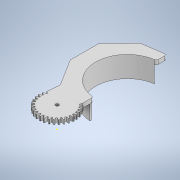
# Autodesk Inventor part: Gripper test sebelah
Saved by Autodesk Inventor 2021 (Build 250183000, 183)
## iProperties
Created: 2025-08-29
Part Number: Gripper test sebelah
Material: Generic
Document SubType Name: Modeling
Designer: Naufal K
Mass: 10.2864 g
Surface Area: 64.4788 cm^2
Volume: 10.2864 cm^3
Density: 1 g/cm^3
Appearance: Default
Author: Naufal K
Autodesk Inventor part; units mm, degrees
ref_plane "YZ Plane" through (0, 0, 0) normal (1, 0, 0) x (0, 1, 0)
ref_plane "XZ Plane" through (0, 0, 0) normal (0, 1, 0) x (-1, 0, 0)
ref_plane "XY Plane" through (0, 0, 0) normal (0, 0, 1) x (1, 0, 0)
sketch "Sketch1" plane through (0, 0, 0) normal (0, 1, 0) x (-1, 0, 0)
  arc A0 (-17.5, 0) -> (-15.9835, -7.1258) centre (0, 0) ccw
  line L0 (14.9666, 1) -> (17.4123, 0.5159)
  line L1 (17.4123, -0.5159) -> (14.9666, -1)
  line L2 (17.4929, 0.4179) -> (17.4929, -0.4179)
  line L3 (17.5, 0) -> (17.4929, 0)
  arc A1 (17.4929, 0.4179) -> (17.4123, 0.5159) centre (17.3929, 0.4179) ccw
  arc A2 (17.4123, -0.5159) -> (17.4929, -0.4179) centre (17.3929, -0.4179) ccw
  line L4 (14.459, 3.9923) -> (16.952, 4.0105)
  arc A3 (17.0507, 3.9306) -> (16.952, 4.0105) centre (16.9527, 3.9105) ccw
  line L5 (17.0507, 3.9306) -> (17.2189, 3.112)
  arc A4 (17.1597, 2.9997) -> (17.2189, 3.112) centre (17.1209, 3.0919) ccw
  line L6 (17.1597, 2.9997) -> (14.8616, 2.0332)
  line L7 (13.3593, 6.8211) -> (15.7977, 7.3408)
  arc A5 (15.9104, 7.2824) -> (15.7977, 7.3408) centre (15.8185, 7.243) ccw
  line L8 (15.9104, 7.2824) -> (16.24, 6.5144)
  arc A6 (16.2046, 6.3925) -> (16.24, 6.5144) centre (16.1481, 6.475) ccw
  line L9 (16.2046, 6.3925) -> (14.1481, 4.9832)
  line L10 (11.7128, 9.3707) -> (13.9966, 10.3705)
  arc A7 (14.1188, 10.3361) -> (13.9966, 10.3705) centre (14.0367, 10.2789) ccw
  line L11 (14.1188, 10.3361) -> (14.5962, 9.6502)
  arc A8 (14.5861, 9.5236) -> (14.5962, 9.6502) centre (14.5141, 9.593) ccw
  line L12 (14.5861, 9.5236) -> (12.8553, 7.7292)
  line L13 (9.5867, 11.5367) -> (11.6225, 12.9758)
  arc A9 (11.7491, 12.9666) -> (11.6225, 12.9758) centre (11.6802, 12.8941) ccw
  line L14 (11.7491, 12.9666) -> (12.3549, 12.3908)
  arc A10 (12.3704, 12.2648) -> (12.3549, 12.3908) centre (12.286, 12.3183) ccw
  line L15 (12.3704, 12.2648) -> (11.0363, 10.1587)
  line L16 (7.0682, 13.2303) -> (8.7726, 15.0497)
  arc A11 (8.8985, 15.0662) -> (8.7726, 15.0497) centre (8.8456, 14.9814) ccw
  line L17 (8.8985, 15.0662) -> (9.6077, 14.6242)
  arc A12 (9.6483, 14.5039) -> (9.6077, 14.6242) centre (9.5548, 14.5393) ccw
  line L18 (9.6483, 14.5039) -> (8.7655, 12.1724)
  line L19 (4.2602, 14.3823) -> (5.5635, 16.5076)
  arc A13 (5.6835, 16.5491) -> (5.5635, 16.5076) centre (5.6488, 16.4553) ccw
  line L20 (5.6835, 16.5491) -> (6.4672, 16.2588)
  arc A14 (6.5312, 16.1492) -> (6.4672, 16.2588) centre (6.4325, 16.1651) ccw
  line L21 (6.5312, 16.1492) -> (6.1357, 13.6877)
  line L22 (1.2779, 14.9455) -> (2.1267, 17.2896)
  arc A15 (2.2359, 17.3544) -> (2.1267, 17.2896) centre (2.2207, 17.2556) ccw
  line L23 (2.2359, 17.3544) -> (3.0619, 17.2279)
  arc A16 (3.1467, 17.1333) -> (3.0619, 17.2279) centre (3.0468, 17.129) ccw
  line L24 (3.1467, 17.1333) -> (3.2548, 14.6426)
  line L25 (-1.7568, 14.8968) -> (-1.3972, 17.3638)
  arc A17 (-1.3033, 17.4492) -> (-1.3972, 17.3638) centre (-1.2982, 17.3494) ccw
  line L26 (-1.3033, 17.4492) -> (-0.4687, 17.4916)
  arc A18 (-0.3666, 17.4161) -> (-0.4687, 17.4916) centre (-0.4636, 17.3917) ccw
  line L27 (-0.3666, 17.4161) -> (0.2407, 14.9981)
  line L28 (-4.7195, 14.2382) -> (-4.8639, 16.7271)
  arc A19 (-4.7891, 16.8297) -> (-4.8639, 16.7271) centre (-4.7641, 16.7329) ccw
  line L29 (-4.7891, 16.8297) -> (-3.9801, 17.0392)
  arc A20 (-3.865, 16.9857) -> (-3.9801, 17.0392) centre (-3.955, 16.9424) ccw
  line L30 (-3.865, 16.9857) -> (-2.7833, 14.7395)
  line L31 (-7.489, 12.9967) -> (-8.1315, 15.4056)
  arc A21 (-8.0789, 15.5211) -> (-8.1315, 15.4056) centre (-8.0349, 15.4314) ccw
  line L32 (-8.0789, 15.5211) -> (-7.3286, 15.8892)
  arc A22 (-7.205, 15.86) -> (-7.3286, 15.8892) centre (-7.2846, 15.7994) ccw
  line L33 (-7.205, 15.86) -> (-5.6934, 13.8775)
  line L34 (-9.9519, 11.2231) -> (-11.0662, 13.4534)
  arc A23 (-11.0379, 13.5772) -> (-11.0662, 13.4534) centre (-10.9767, 13.4981) ccw
  line L35 (-11.0379, 13.5772) -> (-10.3771, 14.0887)
  arc A24 (-10.2502, 14.085) -> (-10.3771, 14.0887) centre (-10.3158, 14.0096) ccw
  line L36 (-10.2502, 14.085) -> (-8.3704, 12.4474)
  line L37 (-12.0074, 8.9901) -> (-13.5478, 10.9504)
  arc A25 (-13.545, 11.0773) -> (-13.5478, 10.9504) centre (-13.4691, 11.0122) ccw
  line L38 (-13.545, 11.0773) -> (-13.0007, 11.7114)
  arc A26 (-12.8756, 11.7334) -> (-13.0007, 11.7114) centre (-12.9248, 11.6463) ccw
  line L39 (-12.8756, 11.7334) -> (-10.7047, 10.5076)
  line L40 (-13.5713, 6.389) -> (-15.4748, 7.9991)
  arc A27 (-15.4976, 8.124) -> (-15.4748, 7.9991) centre (-15.4102, 8.0754) ccw
  line L41 (-15.4976, 8.124) -> (-15.092, 8.8547)
  arc A28 (-14.974, 8.9013) -> (-15.092, 8.8547) centre (-15.0046, 8.8061) ccw
  line L42 (-14.974, 8.9013) -> (-12.6007, 8.1377)
  line L43 (-14.5796, 3.5263) -> (-16.7682, 4.7203)
  arc A29 (-16.8157, 4.838) -> (-16.7682, 4.7203) centre (-16.7203, 4.8081) ccw
  line L44 (-16.8157, 4.838) -> (-16.5655, 5.6354)
  arc A30 (-16.4593, 5.7049) -> (-16.5655, 5.6354) centre (-16.4701, 5.6055) ccw
  line L45 (-16.4593, 5.7049) -> (-13.9809, 5.4346)
  line L46 (-14.991, 0.5193) -> (-17.3751, 1.2483)
  arc A31 (-17.4454, 1.354) -> (-17.3751, 1.2483) centre (-17.3459, 1.3439) ccw
  line L47 (-17.4454, 1.354) -> (-17.3608, 2.1854)
  arc A32 (-17.2707, 2.2749) -> (-17.3608, 2.1854) centre (-17.2613, 2.1753) ccw
  line L48 (-17.2707, 2.2749) -> (-14.7887, 2.509)
  line L49 (-14.7887, -2.509) -> (-17.2707, -2.2749)
  arc A33 (-17.3608, -2.1854) -> (-17.2707, -2.2749) centre (-17.2613, -2.1753) ccw
  line L50 (-17.3608, -2.1854) -> (-17.4454, -1.354)
  arc A34 (-17.3751, -1.2483) -> (-17.4454, -1.354) centre (-17.3459, -1.3439) ccw
  line L51 (-17.3751, -1.2483) -> (-14.991, -0.5193)
  line L52 (-13.9809, -5.4346) -> (-16.4593, -5.7049)
  arc A35 (-16.5655, -5.6354) -> (-16.4593, -5.7049) centre (-16.4701, -5.6055) ccw
  line L53 (-16.5655, -5.6354) -> (-16.8157, -4.838)
  arc A36 (-16.7682, -4.7203) -> (-16.8157, -4.838) centre (-16.7203, -4.8081) ccw
  line L54 (-16.7682, -4.7203) -> (-14.5796, -3.5263)
  line L55 (-12.6007, -8.1377) -> (-14.974, -8.9013)
  arc A37 (-15.092, -8.8547) -> (-14.974, -8.9013) centre (-15.0046, -8.8061) ccw
  line L56 (-15.092, -8.8547) -> (-15.4976, -8.124)
  arc A38 (-15.4748, -7.9991) -> (-15.4976, -8.124) centre (-15.4102, -8.0754) ccw
  line L57 (-15.4748, -7.9991) -> (-13.5713, -6.389)
  line L58 (-10.7047, -10.5076) -> (-12.8756, -11.7334)
  arc A39 (-13.0007, -11.7114) -> (-12.8756, -11.7334) centre (-12.9248, -11.6463) ccw
  line L59 (-13.0007, -11.7114) -> (-13.545, -11.0773)
  arc A40 (-13.5478, -10.9504) -> (-13.545, -11.0773) centre (-13.4691, -11.0122) ccw
  line L60 (-13.5478, -10.9504) -> (-12.0074, -8.9901)
  line L61 (-8.3704, -12.4474) -> (-10.2502, -14.085)
  arc A41 (-10.3771, -14.0887) -> (-10.2502, -14.085) centre (-10.3158, -14.0096) ccw
  line L62 (-10.3771, -14.0887) -> (-11.0379, -13.5772)
  arc A42 (-11.0662, -13.4534) -> (-11.0379, -13.5772) centre (-10.9767, -13.4981) ccw
  line L63 (-11.0662, -13.4534) -> (-9.9519, -11.2231)
  line L64 (-5.6934, -13.8775) -> (-7.205, -15.86)
  arc A43 (-7.3286, -15.8892) -> (-7.205, -15.86) centre (-7.2846, -15.7994) ccw
  line L65 (-7.3286, -15.8892) -> (-8.0789, -15.5211)
  arc A44 (-8.1315, -15.4056) -> (-8.0789, -15.5211) centre (-8.0349, -15.4314) ccw
  line L66 (-8.1315, -15.4056) -> (-7.489, -12.9967)
  line L67 (-2.7833, -14.7395) -> (-3.865, -16.9857)
  arc A45 (-3.9801, -17.0392) -> (-3.865, -16.9857) centre (-3.955, -16.9424) ccw
  line L68 (-3.9801, -17.0392) -> (-4.7891, -16.8297)
  arc A46 (-4.8639, -16.7271) -> (-4.7891, -16.8297) centre (-4.7641, -16.7329) ccw
  line L69 (-4.8639, -16.7271) -> (-4.7195, -14.2382)
  line L70 (0.2407, -14.9981) -> (-0.3666, -17.4161)
  arc A47 (-0.4687, -17.4916) -> (-0.3666, -17.4161) centre (-0.4636, -17.3917) ccw
  line L71 (-0.4687, -17.4916) -> (-1.3033, -17.4492)
  arc A48 (-1.3972, -17.3638) -> (-1.3033, -17.4492) centre (-1.2982, -17.3494) ccw
  line L72 (-1.3972, -17.3638) -> (-1.7568, -14.8968)
  line L73 (3.2548, -14.6426) -> (3.1467, -17.1333)
  arc A49 (3.0619, -17.2279) -> (3.1467, -17.1333) centre (3.0468, -17.129) ccw
  line L74 (3.0619, -17.2279) -> (2.2359, -17.3544)
  arc A50 (2.1267, -17.2896) -> (2.2359, -17.3544) centre (2.2207, -17.2556) ccw
  line L75 (2.1267, -17.2896) -> (1.2779, -14.9455)
  line L76 (6.1357, -13.6877) -> (6.5312, -16.1492)
  arc A51 (6.4672, -16.2588) -> (6.5312, -16.1492) centre (6.4325, -16.1651) ccw
  line L77 (6.4672, -16.2588) -> (5.6835, -16.5491)
  arc A52 (5.5635, -16.5076) -> (5.6835, -16.5491) centre (5.6488, -16.4553) ccw
  line L78 (5.5635, -16.5076) -> (4.2602, -14.3823)
  line L79 (8.7655, -12.1724) -> (9.6483, -14.5039)
  arc A53 (9.6077, -14.6242) -> (9.6483, -14.5039) centre (9.5548, -14.5393) ccw
  line L80 (9.6077, -14.6242) -> (8.8985, -15.0662)
  arc A54 (8.7726, -15.0497) -> (8.8985, -15.0662) centre (8.8456, -14.9814) ccw
  line L81 (8.7726, -15.0497) -> (7.0682, -13.2303)
  line L82 (11.0363, -10.1587) -> (12.3704, -12.2648)
  arc A55 (12.3549, -12.3908) -> (12.3704, -12.2648) centre (12.286, -12.3183) ccw
  line L83 (12.3549, -12.3908) -> (11.7491, -12.9666)
  arc A56 (11.6225, -12.9758) -> (11.7491, -12.9666) centre (11.6802, -12.8941) ccw
  line L84 (11.6225, -12.9758) -> (9.5867, -11.5367)
  line L85 (12.8553, -7.7292) -> (14.5861, -9.5236)
  arc A57 (14.5962, -9.6502) -> (14.5861, -9.5236) centre (14.5141, -9.593) ccw
  line L86 (14.5962, -9.6502) -> (14.1188, -10.3361)
  arc A58 (13.9966, -10.3705) -> (14.1188, -10.3361) centre (14.0367, -10.2789) ccw
  line L87 (13.9966, -10.3705) -> (11.7128, -9.3707)
  line L88 (14.1481, -4.9832) -> (16.2046, -6.3925)
  arc A59 (16.24, -6.5144) -> (16.2046, -6.3925) centre (16.1481, -6.475) ccw
  line L89 (16.24, -6.5144) -> (15.9104, -7.2824)
  arc A60 (15.7977, -7.3408) -> (15.9104, -7.2824) centre (15.8185, -7.243) ccw
  line L90 (15.7977, -7.3408) -> (13.3593, -6.8211)
  line L91 (14.8616, -2.0332) -> (17.1597, -2.9997)
  arc A61 (17.2189, -3.112) -> (17.1597, -2.9997) centre (17.1209, -3.0919) ccw
  line L92 (17.2189, -3.112) -> (17.0507, -3.9306)
  arc A62 (16.952, -4.0105) -> (17.0507, -3.9306) centre (16.9527, -3.9105) ccw
  line L93 (16.952, -4.0105) -> (14.459, -3.9923)
  arc A63 (14.459, 3.9923) -> (14.1481, 4.9832) centre (0, 0) ccw
  arc A64 (13.3593, 6.8211) -> (12.8553, 7.7292) centre (0, 0) ccw
  arc A65 (11.7128, 9.3707) -> (11.0363, 10.1587) centre (0, 0) ccw
  arc A66 (9.5867, 11.5367) -> (8.7655, 12.1724) centre (0, 0) ccw
  arc A67 (7.0682, 13.2303) -> (6.1357, 13.6877) centre (0, 0) ccw
  arc A68 (4.2602, 14.3823) -> (3.2548, 14.6426) centre (0, 0) ccw
  arc A69 (1.2779, 14.9455) -> (0.2407, 14.9981) centre (0, 0) ccw
  arc A70 (-1.7568, 14.8968) -> (-2.7833, 14.7395) centre (0, 0) ccw
  arc A71 (-4.7195, 14.2382) -> (-5.6934, 13.8775) centre (0, 0) ccw
  arc A72 (-7.489, 12.9967) -> (-8.3704, 12.4474) centre (0, 0) ccw
  arc A73 (-9.9519, 11.2231) -> (-10.7047, 10.5076) centre (0, 0) ccw
  arc A74 (-12.0074, 8.9901) -> (-12.6007, 8.1377) centre (0, 0) ccw
  arc A75 (-13.5713, 6.389) -> (-13.9809, 5.4346) centre (0, 0) ccw
  arc A76 (-14.5796, 3.5263) -> (-14.7887, 2.509) centre (0, 0) ccw
  arc A77 (-14.991, 0.5193) -> (-14.991, -0.5193) centre (0, 0) ccw
  arc A78 (-14.7887, -2.509) -> (-14.5796, -3.5263) centre (0, 0) ccw
  arc A79 (-13.9809, -5.4346) -> (-13.5713, -6.389) centre (0, 0) ccw
  arc A80 (-12.6007, -8.1377) -> (-12.0074, -8.9901) centre (0, 0) ccw
  arc A81 (-10.7047, -10.5076) -> (-9.9519, -11.2231) centre (0, 0) ccw
  arc A82 (-8.3704, -12.4474) -> (-7.489, -12.9967) centre (0, 0) ccw
  arc A83 (-5.6934, -13.8775) -> (-4.7195, -14.2382) centre (0, 0) ccw
  arc A84 (-2.7833, -14.7395) -> (-1.7568, -14.8968) centre (0, 0) ccw
  arc A85 (0.2407, -14.9981) -> (1.2779, -14.9455) centre (0, 0) ccw
  arc A86 (3.2548, -14.6426) -> (4.2602, -14.3823) centre (0, 0) ccw
  arc A87 (6.1357, -13.6877) -> (7.0682, -13.2303) centre (0, 0) ccw
  arc A88 (8.7655, -12.1724) -> (9.5867, -11.5367) centre (0, 0) ccw
  arc A89 (11.0363, -10.1587) -> (11.7128, -9.3707) centre (0, 0) ccw
  arc A90 (12.8553, -7.7292) -> (13.3593, -6.8211) centre (0, 0) ccw
  arc A91 (14.1481, -4.9832) -> (14.459, -3.9923) centre (0, 0) ccw
  arc A92 (14.8616, -2.0332) -> (14.9666, -1) centre (0, 0) ccw
  arc A93 (14.9666, 1) -> (14.8616, 2.0332) centre (0, 0) ccw
  arc A94 (-10.7047, -83.8219) -> (-10.7047, -23.8219) centre (-10.7047, -53.8219) ccw
  line L94 (-10.7047, -83.8219) -> (-10.7047, -93.8219)
  line L95 (-10.7047, -93.8219) -> (11.3814, -90.5076)
  line L96 (11.3814, -90.5076) -> (30.7761, -70.2991)
  line L97 (30.7761, -70.2991) -> (30.7761, -43.252)
  line L98 (30.7761, -43.252) -> (14.923, -18.0076)
  line L99 (14.923, -18.0076) -> (15.9104, -7.2824)
  line L100 (-10.7047, -23.8219) -> (-10.7047, -10.5076)
  point P0 (17.1348, 3.5213)
  point P1 (-14.2219, -10.1974)
  point P2 (16.0752, 6.8984)
  point P3 (-11.8781, -12.8515)
  point P4 (14.3575, 9.9931)
  point P5 (-9.048, -14.9795)
  point P6 (12.052, 12.6787)
  point P7 (-5.8474, -16.4942)
  point P8 (9.2531, 14.8452)
  point P9 (-2.4075, -17.3336)
  point P10 (6.0754, 16.404)
  point P11 (1.131, -17.4634)
  point P12 (2.6489, 17.2911)
  point P13 (4.6232, -16.8783)
  point P14 (-0.886, 17.4704)
  point P15 (7.9262, -15.6021)
  point P16 (-4.3846, 16.9344)
  point P17 (10.9046, -13.6872)
  point P18 (-7.7038, 15.7052)
  point P19 (13.4366, -11.2119)
  point P20 (-10.7075, 13.8329)
  point P21 (15.4185, -8.2777)
  point P22 (-13.2728, 11.3944)
  point P23 (16.7692, -5.0045)
  point P24 (-15.2948, 8.4893)
  point P25 (17.4333, -1.5264)
  point P26 (-16.6906, 5.2367)
  point P27 (17.3837, 2.0141)
  point P28 (-17.4031, 1.7697)
  point P29 (16.6224, 5.4722)
  point P30 (-17.4031, -1.7697)
  point P31 (15.1806, 8.7062)
  point P32 (-16.6906, -5.2367)
  point P33 (13.1173, 11.5839)
  point P34 (-15.2948, -8.4893)
  point P35 (10.517, 13.9872)
  point P36 (-13.2728, -11.3944)
  point P37 (7.4861, 15.818)
  point P38 (-10.7075, -13.8329)
  point P39 (4.1487, 17.0011)
  point P40 (-7.7038, -15.7052)
  point P41 (0.6415, 17.4882)
  point P42 (-4.3846, -16.9344)
  point P43 (-2.892, 17.2594)
  point P44 (-0.886, -17.4704)
  point P45 (-6.3071, 16.3239)
  point P46 (2.6489, -17.2911)
  point P47 (-9.4639, 14.7202)
  point P48 (6.0754, -16.404)
  point P49 (-12.2334, 12.5138)
  point P50 (9.2531, -14.8452)
  point P51 (-14.502, 9.7951)
  point P52 (12.052, -12.6787)
  point P53 (-16.1768, 6.6753)
  point P54 (14.3575, -9.9931)
  point P55 (-17.1894, 3.2823)
  point P56 (16.0752, -6.8984)
  point P57 (-17.4983, -0.2451)
  point P58 (17.1348, -3.5213)
  point P59 (-17.0908, -3.7624)
  point P60 (-10.7047, -13.8351)
  dimension "d1" = 35
  dimension "d6" = 0.1
  dimension "d9" = 360
  dimension "d13" = 60
  dimension "d14" = 30
  dimension "d15" = 10
  constraints: 202 end point, 128 point on circle, 64 centre point, 32 point on line, 31 midpoint, 4 tangent, 3 vertical, 1 equal radius, 1 horizontal, 1 vertical alignment, 560 other
  measures "d1" diameter of A0
  measures "d6" radius of A1
  measures "d13" distance of L100.start L94.start
  measures "d14" radius of A94
  measures "d15" distance of L94.start L94.end
extrude "Extrusion1" add sketch "Sketch1" along normal blind 4 contours L0 A1 L2 A2 L1 A92 L91 A61 L92 A62 L93 A91 L88 A59 L89 A60 L90 A90 L85 A57 L86 A58 L87 A89 L82 A55 L83 A56 L84 A88 L79 A53 L80 A54 L81 A87 L76 A51 L77 A52 L78 A86 L73 A49 L74 A50 L75 A85 L70 A47 L71 A48 L72 A84 L67 A45 L68 A46 L69 A83 L64 A43 L65 A44 L66 A82 L61 A41 L62 L100 L63 A81 L58 A39 L59 A40 L60 A80 L55 A37 L56 A38 L57 A79 L52 A35 L53 A36 L54 A78 L49 A33 L50 A34 L51 A77 L46 A31 L47 A32 L48 A76 L43 A29 L44 A30 L45 A75 L40 A27 L41 A28 L42 A74 L37 A25 L38 A26 L39 A73 L34 A23 L35 A24 L36 A72 L31 A21 L32 A22 L33 A71 L28 A19 L29 A20 L30 A70 L25 A17 L26 A18 L27 A69 L22 A15 L23 A16 L24 A68 L19 A13 L20 A14 L21 A67 L16 A11 L17 A12 L18 A66 L13 A9 L14 A10 L15 A65 L10 A7 L11 A8 L12 A64 L7 A5 L8 A6 L9 A63 L4 A3 L5 A4 L6 A93 | L99 L98 L97 L96 L95 L94 A94 L100 L62 A41 L61 A82 L66 A44 L65 A43 L64 A83 L69 A46 L68 A45 L67 A84 L72 A48 L71 A47 L70 A85 L75 A50 L74 A49 L73 A86 L78 A52 L77 A51 L76 A87 L81 A54 L80 A53 L79 A88 L84 A56 L83 A55 L82 A89 L87 A58 L86 A57 L85 A90 L90 A60 | L62 A42 L63 L100
sketch "Sketch4" plane through (0, 4, 0) normal (0, 1, 0) x (1, 0, 0)
  circle A0 centre (0, 0) radius 1.5
  dimension "d29" = 3
  constraints: 1 centre point, 1 coincident
  measures "d29" diameter of A0
extrude "Extrusion4" cut sketch "Sketch4" against normal blind 10
sketch "Sketch6" plane through (0, 4, 0) normal (0, 1, 0) x (1, 0, 0)
  arc A0 (8.8297, 85.3519) -> (8.8297, 22.4512) centre (10.9908, 53.9015) ccw
  line L0 (8.8297, 85.3519) -> (8.8297, 83.7632)
  line L1 (8.8297, 22.4512) -> (8.8297, 23.8805)
  arc A1 (8.8297, 83.7632) -> (8.8297, 23.8805) centre (13.1903, 53.8219) ccw
  point P0 (0, 0)
  constraints: 4 end point, 4 point on circle, 2 centre point, 1 collinear, 1 vertical
extrude "Extrusion6" add sketch "Sketch6" against normal blind 20
sketch "Sketch10" plane through (0, 4, 0) normal (0, 1, 0) x (1, 0, 0)
  line L0 (8.4079, 93.4772) -> (2.4719, 133.0343) projected
  circle A0 centre (5.4399, 112.1899) radius 11
  point P0 (0, 0)
  point P1 (3.9641, 123.0905)
  point P2 (7.2285, 101.3363)
  dimension "d43" = 22
  constraints: 1 centre point
  measures "d43" diameter of A0
extrude "Extrusion9" cut sketch "Sketch10" against normal blind 5 contours A0 L0 picked at (4.3754, 108.7301)
fillet "Fillet11" radius 2 3 edges at (-30.7761, 2, -43.252) (-30.7761, 2, -70.2991) (-11.3814, 2, -90.5076)
fillet "Fillet12" radius 2 1 edges at (-14.923, 2, -18.0076)
fillet "Fillet13" radius 2 1 edges at (10.7047, 2, -23.8219)
fillet "Fillet14" radius 2 3 edges at (10.7047, 2, -93.8219) (10.7047, 2, -83.8219) (8.8297, -8, -85.3519)
sketch "Sketch18" plane through (0, -16, 0) normal (0, -1, 0) x (1, 0, 0)
  point P0 (0, 0)
sketch "Sketch12" plane through (0, 4, 0) normal (0, 1, 0) x (1, 0, 0)
  line L0 (10.7047, 93.8219) -> (-11.3814, 90.5076) projected
  line L1 (10.7047, 93.8219) -> (10.7047, 133.8219)
  line L2 (10.7047, 133.8219) -> (-11.3814, 133.8219)
  line L3 (-11.3814, 133.8219) -> (-11.3814, 90.5076)
  line L4 (-11.3814, 90.5076) -> (10.7047, 93.8219)
  point P0 (0, 0)
  dimension "d46" = 40
  constraints: 8 end point, 2 perpendicular, 1 collinear, 1 vertical
  measures "d46" distance of L0.start L1.end
sketch "Sketch13" plane through (0, 4, 0) normal (0, 1, 0) x (1, 0, 0)
  line L0 (10.7047, 83.8219) -> (10.7047, 133.8219) projected
  circle A0 centre (10.7047, 108.8219) radius 20
  point P0 (0, 0)
  point P1 (10.7047, 128.8219)
  point P2 (10.7047, 88.8219)
  dimension "d49" = 40
  constraints: 1 centre point, 1 midpoint
  measures "d49" diameter of A0
sketch "Sketch15" plane through (0, 4, 0) normal (0, 1, 0) x (1, 0, 0)
  arc A0 (9.6186, 133.8219) -> (-11.3814, 112.8219) centre (9.6186, 112.8219) ccw projected
  line L0 (-11.3814, 112.8219) -> (-24.972, 76.3467)
  line L1 (-11.3814, 90.5076) -> (-30.7761, 70.2991) projected
  line L2 (-11.3814, 90.5076) -> (-24.972, 76.3467)
  line L3 (-11.3814, 90.5076) -> (-11.3814, 112.8219) projected
  line L4 (-11.3814, 90.5076) -> (-11.3814, 112.8219)
  point P0 (0, 0)
  constraints: 6 end point, 3 point on line, 1 collinear
sketch "Sketch16" plane through (0, 4, 0) normal (0, 1, 0) x (1, 0, 0)
  arc A0 (8.6085, 133.7976) -> (-10.3552, 119.3061) centre (9.6186, 112.8219) ccw projected
  line L0 (7.142, 133.6753) -> (7.8607, 128.309)
  line L1 (7.8607, 128.309) -> (13.4517, 129.2923)
  line L2 (13.4517, 129.2923) -> (10.9454, 136.522)
  line L3 (10.9454, 136.522) -> (7.142, 133.6753)
  point P0 (0, 0)
  constraints: 8 end point, 1 point on circle
sketch "Sketch17" plane through (0, 4, 0) normal (0, 1, 0) x (1, 0, 0)
  arc A0 (8.8865, 128.7391) -> (8.8865, 88.9047) centre (10.7047, 108.8219) ccw projected
  arc A1 (5.8551, 128.225) -> (8.8865, 88.9047) centre (10.7047, 108.8219) ccw
  arc A2 (5.8551, 129.1895) -> (8.8865, 87.4937) centre (10.724, 108.5854) ccw
  line L0 (5.8551, 129.1895) -> (5.8551, 128.225)
  line L1 (8.8865, 88.9047) -> (8.8865, 87.4937)
  point P0 (0, 0)
  constraints: 4 end point, 4 point on circle, 2 centre point, 1 concentric, 1 parallel, 1 vertical
sketch "Sketch5" plane through (0, 0, 0) normal (0, -1, 0) x (1, 0, 0)
  arc A0 (10.7044, -87.4131) -> (10.7629, -127.407) centre (10.3866, -107.4106) ccw
  line L0 (10.7629, -127.407) -> (10.7629, -131.7181)
  line L1 (10.7629, -131.7181) -> (-2.3786, -126.5219)
  line L2 (-2.3786, -126.5219) -> (-11.9395, -115.5549)
  line L3 (-11.9395, -115.5549) -> (-11.9395, -95.8422)
  line L4 (-11.9395, -95.8422) -> (-10.6703, -93.5029)
  line L5 (8.0611, -83.6994) -> (10.7044, -87.4131)
  line L6 (-10.6703, -93.5029) -> (-4.0081, -81.3331)
  arc A1 (10.7047, -23.8219) -> (10.7047, -83.8219) centre (10.7047, -53.8219) ccw projected
  arc A2 (-3.4327, -80.282) -> (8.0611, -83.6994) centre (10.6543, -53.9409) ccw
  line L7 (-3.4327, -80.282) -> (-4.0081, -81.3331)
  point P0 (0, 0)
  point P1 (8.8297, -23.8805)
  point P2 (8.8297, -83.7632)
  point P3 (8.0655, -83.7056)
  point P4 (1.5447, -82.3892)
  point P5 (-3.4327, -80.282)
  dimension "d32" = 40
  constraints: 16 end point, 6 point on circle, 2 centre point, 1 parallel, 1 vertical
  measures "d32" diameter of A0
sketch "Sketch2" plane through (0, 4, 0) normal (0, 1, 0) x (1, 0, 0)
  arc A0 (-4.8589, 1.1794) -> (4.7697, 1.4999) centre (0, 0) ccw
  line L0 (5, 0) -> (2.28, 17.7167)
  line L1 (0.3031, 19.4132) -> (-0.9027, 19.4132)
  line L2 (-2.8886, 17.6508) -> (-5, 0)
  arc A1 (-2.589, 19.4132) -> (-2.6883, 19.3251) centre (-2.589, 19.3132) ccw
  arc A2 (-0.9027, 19.4132) -> (-2.8886, 17.6508) centre (-0.9027, 17.4132) ccw
  arc A3 (2.28, 17.7167) -> (0.3031, 19.4132) centre (0.3031, 17.4132) ccw
  dimension "d22" = 10
  dimension "d23" = 0.1
  dimension "d24" = 2
  constraints: 10 point on circle, 6 end point, 6 tangent, 4 centre point, 4 point on line, 1 coincident, 1 equal radius, 1 horizontal
  measures "d22" diameter of A0
  measures "d23" radius of A1
  measures "d24" radius of A2
sketch "Sketch3" plane through (0, 2, 0) normal (0, 1, 0) x (1, 0, 0)
  circle A0 centre (0, 0) radius 3.2728
  constraints: 1 centre point, 1 coincident
body "Solid1"
